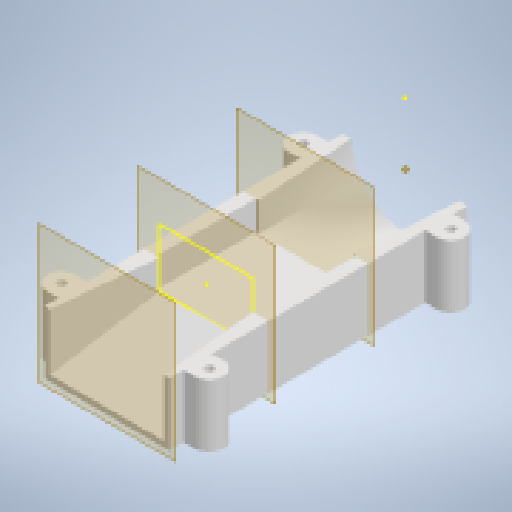
# Autodesk Inventor part: heater_case_bottom
Saved by Autodesk Inventor 2025.4 (Build 294407000, 407)
## iProperties
Created: 2025-12-17
Part Number: heater_case_bottom
Material: Ogólny
Document SubType Name: Modeling
Designer: FOX
Density: 1 g/cm^3
Appearance: Domyślna
Author: FOX
Autodesk Inventor part; units mm, degrees
ref_plane "YZ Plane" through (0, 0, 0) normal (1, 0, 0) x (0, 1, 0)
ref_plane "XZ Plane" through (0, 0, 0) normal (0, 1, 0) x (-1, 0, 0)
ref_plane "Płaszczyzna konstrukcyjna3" through (0, 0, 35) normal (0, 0, 1) x (1, 0, 0)
ref_plane "Płaszczyzna konstrukcyjna4" through (0, 0, 70) normal (0, 0, 1) x (1, 0, 0)
ref_plane "Płaszczyzna konstrukcyjna5" through (0, 0, 105) normal (0, 0, 1) x (1, 0, 0)
sketch "Szkic7" plane through (0, 0, 0) normal (0, 0, 1) x (1, 0, 0)
  circle A0 centre (0, 0) radius 19
  dimension "d41" = 38
  constraints: 1 centre point, 1 coincident
  measures "d41" diameter of A0
sketch "Szkic9" plane through (0, 0, 35) normal (0, 0, 1) x (1, 0, 0)
  line L0 (16.5, 10.25) -> (-16.5, 10.25)
  line L1 (-16.5, 10.25) -> (-16.5, -10.25)
  line L2 (-16.5, -10.25) -> (16.5, -10.25)
  line L3 (16.5, -10.25) -> (16.5, 10.25)
  line L4 (16.5, 10.25) -> (-16.5, -10.25) construction
  line L5 (-16.5, 10.25) -> (16.5, -10.25) construction
  point P0 (0, 0)
  dimension "d42" = 33
  dimension "d43" = 20.5
  constraints: 12 end point, 2 midpoint, 2 parallel, 1 horizontal, 1 perpendicular
  measures "d42" distance of L2.end L1.end
  measures "d43" distance of L1.end L0.end
sketch "Szkic10" plane through (0, 0, 70) normal (0, 0, 1) x (1, 0, 0)
  line L0 (16.5, 10.25) -> (-16.5, 10.25) projected
  line L1 (-16.5, 10.25) -> (-16.5, -10.25) projected
  line L2 (-16.5, -10.25) -> (16.5, -10.25) projected
  line L3 (16.5, -10.25) -> (16.5, 10.25) projected
  point P0 (0, 0)
sketch "Szkic11" plane through (0, 0, 105) normal (0, 0, 1) x (1, 0, 0)
  line L0 (20, -20) -> (-20, -20)
  line L1 (-20, -20) -> (-20, 20)
  line L2 (-20, 20) -> (20, 20)
  line L3 (20, 20) -> (20, -20)
  line L4 (20, -20) -> (-20, 20) construction
  line L5 (-20, -20) -> (20, 20) construction
  point P0 (0, 0)
  dimension "d44" = 40
  dimension "d45" = 40
  constraints: 12 end point, 2 midpoint, 2 parallel, 1 horizontal, 1 perpendicular
  measures "d44" distance of L1.end L2.end
  measures "d45" distance of L0.end L1.end
sketch "Szkic12" plane through (0, 0, 0) normal (0, 0, 1) x (1, 0, 0)
  line L0 (-22, -22) -> (22, -22)
  line L1 (22, -22) -> (22, 22)
  line L2 (22, 22) -> (-22, 22)
  line L3 (-22, 22) -> (-22, -22)
  line L4 (-22, -22) -> (22, 22) construction
  line L5 (22, -22) -> (-22, 22) construction
  point P0 (0, 0)
  dimension "d46" = 44
  dimension "d47" = 44
  constraints: 12 end point, 2 midpoint, 2 parallel, 1 horizontal, 1 perpendicular
  measures "d46" distance of L2.end L1.end
  measures "d47" distance of L1.end L0.end
extrude "Wyciągnięcie proste1" add sketch "Szkic12" along normal blind 105
extrude "Wyciągnięcie proste2" cut sketch "Szkic9" along normal blind 35
loft "Wyciągnięcie złożone1" cut profiles "Szkic7" section 2 edges at (-16.5, 0, 35) (0, -10.25, 35) (16.5, 0, 35) (0, 10.25, 35)
loft "Wyciągnięcie złożone2" cut profiles "Szkic11" section 2 edges at (-16.5, 0, 70) (0, 10.25, 70) (16.5, 0, 70) (0, -10.25, 70)
sketch "Szkic13" plane through (0, 0, 70) normal (0, 0, 1) x (1, 0, 0)
  line L0 (-17.5, -10.25) -> (17.5, -10.25)
  line L1 (17.5, -10.25) -> (17.5, 10.25)
  line L2 (17.5, 10.25) -> (-17.5, 10.25)
  line L3 (-17.5, 10.25) -> (-17.5, -10.25)
  line L4 (-17.5, -10.25) -> (17.5, 10.25) construction
  line L5 (17.5, -10.25) -> (-17.5, 10.25) construction
  point P0 (0, 0)
  dimension "d60" = 35
  dimension "d61" = 20.5
  constraints: 12 end point, 2 midpoint, 2 parallel, 1 horizontal, 1 perpendicular
  measures "d60" distance of L2.end L1.end
  measures "d61" distance of L1.end L0.end
extrude "Wyciągnięcie proste3" cut sketch "Szkic13" against normal blind 35
sketch "Szkic14" plane through (-22, 22, 0) normal (0, 1, 0) x (1, 0, 0)
  point P0 (22, 0)
sketch "Szkic15" plane through (-16.2734, 10.25, 35) normal (0, -1, 0) x (1, 0, 0)
  line L0 (32.5467, 0) -> (0, 0) construction
  line L1 (16.2734, 0) -> (16.2734, -12) construction
  circle A0 centre (16.2734, -12) radius 4
  point P0 (16.2734, -35)
  dimension "d64" = 12
  dimension "d65" = 8
  constraints: 2 end point, 1 centre point, 1 coincident, 1 midpoint, 1 vertical
  measures "d64" distance of L1.start L1.end
  measures "d65" diameter of A0
extrude "Wyciągnięcie proste4" cut sketch "Szkic15" against normal through all
sketch "Szkic16" plane through (0, 0, 0) normal (0, 0, -1) x (-1, 0, 0)
  line L0 (-16, -16) -> (16, -16) construction
  line L1 (16, -16) -> (16, 16) construction
  line L2 (16, 16) -> (-16, 16) construction
  line L3 (-16, 16) -> (-16, -16) construction
  line L4 (-16, -16) -> (16, 16) construction
  line L5 (16, -16) -> (-16, 16) construction
  circle A0 centre (-16, 16) radius 1.5
  circle A1 centre (-16, -16) radius 1.5
  circle A2 centre (16, -16) radius 1.5
  circle A3 centre (16, 16) radius 1.5
  point P0 (0, 0)
  dimension "d68" = 32
  dimension "d69" = 32
  dimension "d70" = 3
  constraints: 12 end point, 4 centre point, 4 coincident, 3 equal radius, 2 midpoint, 2 parallel, 1 horizontal, 1 perpendicular
  measures "d68" distance of L2.end L1.end
  measures "d69" distance of L1.end L0.end
  measures "d70" diameter of A0
extrude "Wyciągnięcie proste5" cut sketch "Szkic16" against normal blind 10
sketch "Szkic17" plane through (0, 0, 0) normal (0, 1, 0) x (-1, 0, 0)
  line L0 (-35.497, 120.9522) -> (40.1676, 120.9522)
  line L1 (40.1676, 120.9522) -> (40.1676, -13.5628)
  line L2 (40.1676, -13.5628) -> (-35.497, -13.5628)
  line L3 (-35.497, -13.5628) -> (-35.497, 120.9522)
  point P0 (0, 0)
  constraints: 8 end point, 2 parallel, 1 horizontal, 1 perpendicular
sketch "Szkic18" plane through (-22, 22, 0) normal (0, 1, 0) x (1, 0, 0)
  point P0 (22, 0)
sketch "Szkic19" plane through (-22, 22, 0) normal (0, 1, 0) x (1, 0, 0)
  line L0 (44, 0) -> (44, -105) projected
  line L1 (44, -105) -> (44, -95) construction
  line L2 (44, -95) -> (48, -95) construction
  arc A0 (48, -100) -> (48, -90) centre (48, -95) ccw
  line L3 (48, -100) -> (44, -100)
  line L4 (48, -90) -> (44, -90)
  line L5 (44, -100) -> (44, -90)
  line L6 (22, -110.411) -> (22, 7.1772) construction
  line L7 (-9.1147, -52.5) -> (56.3126, -52.5) construction
  line L8 (44, -10) -> (48, -10) construction
  arc A1 (48, -15) -> (48, -5) centre (48, -10) ccw
  line L9 (48, -5) -> (44, -5)
  line L10 (48, -15) -> (44, -15)
  line L11 (44, -5) -> (44, -15)
  line L12 (0, 0) -> (0, -105)
  line L13 (0, -105) -> (0, -95) construction
  line L14 (0, -95) -> (-4, -95) construction
  arc A2 (-4, -90) -> (-4, -100) centre (-4, -95) ccw
  line L15 (-4, -100) -> (0, -100)
  line L16 (-4, -90) -> (0, -90)
  line L17 (0, -100) -> (0, -90)
  line L18 (0, -10) -> (-4, -10) construction
  arc A3 (-4, -5) -> (-4, -15) centre (-4, -10) ccw
  line L19 (-4, -5) -> (0, -5)
  line L20 (-4, -15) -> (0, -15)
  line L21 (0, -5) -> (0, -15)
  point P0 (22, 0)
  dimension "d73" = 10
  dimension "d74" = 4
  dimension "d75" = 10
  constraints: 42 end point, 23 symmetric about line, 8 point on circle, 4 centre point, 4 coincident, 4 point on line, 3 horizontal, 2 midpoint, 2 tangent, 1 collinear, 1 perpendicular, 1 vertical, 3 other
  measures "d73" distance of L0.end L1.end
  measures "d74" distance of L1.end L2.end
  measures "d75" diameter of A0
extrude "Wyciągnięcie proste6" add sketch "Szkic19" against normal up to surface (44 mm away)
sketch "Szkic20" plane through (-22, 22, 0) normal (0, 1, 0) x (1, 0, 0)
  arc A0 (48, -15) -> (48, -5) centre (48, -10) ccw projected
  arc A1 (-4, -5) -> (-4, -15) centre (-4, -10) ccw projected
  arc A2 (-4, -90) -> (-4, -100) centre (-4, -95) ccw projected
  arc A3 (48, -100) -> (48, -90) centre (48, -95) ccw projected
  point P0 (22, 0)
  constraints: 4 coincident
hole "Otwór1" at (26, 22, 10) at (-26, 22, 10) at (26, 22, 95) at (-26, 22, 95) direction (0, -1, 0) diameter 3 end through all counterbore diameter 5 counterbore depth 2
extrude "Wyciągnięcie proste7" cut sketch "Szkic17" along normal up to surface (22 mm away)
